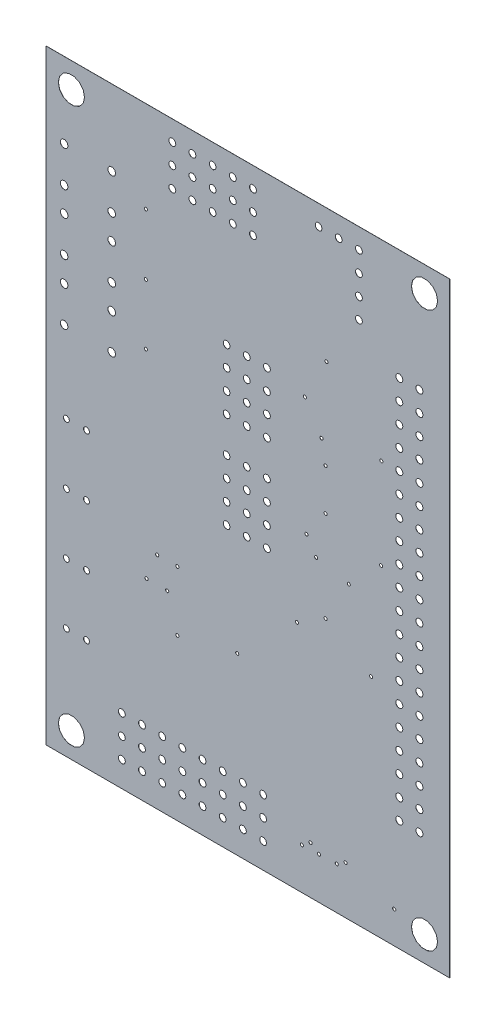
# Autodesk Inventor part: quick-start-plus_Outline4
Saved by Autodesk Inventor 2013 (Build 170138000, 138)
## iProperties
Created: 2013-01-27
Part Number: quick-start-plus_Outline4
Material: Generic
Document SubType Name: Modeling
Designer: davidgitz
Density: 1 g/cm^3
Author: davidgitz
Autodesk Inventor part; units mm, degrees
ref_plane "YZ Plane" through (0, 0, 0) normal (1, 0, 0) x (0, 1, 0)
ref_plane "XZ Plane" through (0, 0, 0) normal (0, 1, 0) x (-1, 0, 0)
ref_plane "XY Plane" through (0, 0, 0) normal (0, 0, 1) x (1, 0, 0)
sketch "Sketch1" plane through (0, 0, 0) normal (0, 0, 1) x (1, 0, 0)
  line L0 (203.2, 203.2) -> (254, 203.2)
  line L1 (254, 203.2) -> (254, 279.4)
  line L2 (254, 279.4) -> (203.2, 279.4)
  line L3 (203.2, 279.4) -> (203.2, 203.2)
  circle A0 centre (236.474, 209.1944) radius 0.2032
  circle A1 centre (227.2538, 225.2218) radius 0.2032
  circle A2 centre (219.71, 223.393) radius 0.2032
  circle A3 centre (237.1852, 240.6396) radius 0.2032
  circle A4 centre (238.379, 251.2314) radius 0.2032
  circle A5 centre (238.4806, 262.636) radius 0.2032
  circle A6 centre (237.871, 253.9746) radius 0.2032
  circle A7 centre (245.3894, 255.27) radius 0.2032
  circle A8 centre (245.364, 243.84) radius 0.2032
  circle A9 centre (235.966, 242.57) radius 0.2032
  circle A10 centre (234.7722, 232.3592) radius 0.2032
  circle A11 centre (244.094, 231.1146) radius 0.2032
  circle A12 centre (217.17, 230.9114) radius 0.2032
  circle A13 centre (219.71, 230.9114) radius 0.2032
  circle A14 centre (247.015, 207.2132) radius 0.2032
  circle A15 centre (215.7476, 267.8938) radius 0.2032
  circle A16 centre (215.7476, 260.223) radius 0.2032
  circle A17 centre (215.7476, 252.6284) radius 0.2032
  circle A18 centre (241.3, 239.776) radius 0.2032
  circle A19 centre (238.379, 234.569) radius 0.2032
  circle A20 centre (238.379, 246.0244) radius 0.2032
  circle A21 centre (235.7628, 257.429) radius 0.2032
  circle A22 centre (215.8238, 227.6602) radius 0.2032
  circle A23 centre (218.44, 227.6348) radius 0.2032
  circle A24 centre (240.8936, 209.2198) radius 0.2032
  circle A25 centre (239.776, 208.534) radius 0.2032
  circle A26 centre (237.5408, 208.4578) radius 0.2032
  circle A27 centre (235.3818, 208.407) radius 0.2032
  circle A28 centre (212.725, 211.455) radius 0.4445
  circle A29 centre (212.725, 208.915) radius 0.4445
  circle A30 centre (212.725, 206.375) radius 0.4445
  circle A31 centre (215.265, 211.455) radius 0.4445
  circle A32 centre (215.265, 208.915) radius 0.4445
  circle A33 centre (215.265, 206.375) radius 0.4445
  circle A34 centre (217.805, 211.455) radius 0.4445
  circle A35 centre (217.805, 208.915) radius 0.4445
  circle A36 centre (217.805, 206.375) radius 0.4445
  circle A37 centre (220.345, 211.455) radius 0.4445
  circle A38 centre (220.345, 208.915) radius 0.4445
  circle A39 centre (220.345, 206.375) radius 0.4445
  circle A40 centre (222.885, 211.455) radius 0.4445
  circle A41 centre (222.885, 208.915) radius 0.4445
  circle A42 centre (222.885, 206.375) radius 0.4445
  circle A43 centre (225.425, 211.455) radius 0.4445
  circle A44 centre (225.425, 208.915) radius 0.4445
  circle A45 centre (225.425, 206.375) radius 0.4445
  circle A46 centre (227.965, 211.455) radius 0.4445
  circle A47 centre (227.965, 208.915) radius 0.4445
  circle A48 centre (227.965, 206.375) radius 0.4445
  circle A49 centre (230.505, 211.455) radius 0.4445
  circle A50 centre (230.505, 208.915) radius 0.4445
  circle A51 centre (230.505, 206.375) radius 0.4445
  circle A52 centre (237.49, 276.86) radius 0.4445
  circle A53 centre (240.03, 276.86) radius 0.4445
  circle A54 centre (247.65, 265.43) radius 0.4572
  circle A55 centre (247.65, 262.89) radius 0.4572
  circle A56 centre (247.65, 260.35) radius 0.4572
  circle A57 centre (247.65, 257.81) radius 0.4572
  circle A58 centre (247.65, 255.27) radius 0.4572
  circle A59 centre (247.65, 252.73) radius 0.4572
  circle A60 centre (247.65, 250.19) radius 0.4572
  circle A61 centre (247.65, 247.65) radius 0.4572
  circle A62 centre (247.65, 245.11) radius 0.4572
  circle A63 centre (247.65, 242.57) radius 0.4572
  circle A64 centre (247.65, 240.03) radius 0.4572
  circle A65 centre (247.65, 237.49) radius 0.4572
  circle A66 centre (247.65, 234.95) radius 0.4572
  circle A67 centre (247.65, 232.41) radius 0.4572
  circle A68 centre (247.65, 229.87) radius 0.4572
  circle A69 centre (247.65, 227.33) radius 0.4572
  circle A70 centre (247.65, 224.79) radius 0.4572
  circle A71 centre (247.65, 222.25) radius 0.4572
  circle A72 centre (247.65, 219.71) radius 0.4572
  circle A73 centre (247.65, 217.17) radius 0.4572
  circle A74 centre (250.19, 217.17) radius 0.4572
  circle A75 centre (250.19, 219.71) radius 0.4572
  circle A76 centre (250.19, 222.25) radius 0.4572
  circle A77 centre (250.19, 224.79) radius 0.4572
  circle A78 centre (250.19, 227.33) radius 0.4572
  circle A79 centre (250.19, 229.87) radius 0.4572
  circle A80 centre (250.19, 232.41) radius 0.4572
  circle A81 centre (250.19, 234.95) radius 0.4572
  circle A82 centre (250.19, 237.49) radius 0.4572
  circle A83 centre (250.19, 240.03) radius 0.4572
  circle A84 centre (250.19, 242.57) radius 0.4572
  circle A85 centre (250.19, 245.11) radius 0.4572
  circle A86 centre (250.19, 247.65) radius 0.4572
  circle A87 centre (250.19, 250.19) radius 0.4572
  circle A88 centre (250.19, 252.73) radius 0.4572
  circle A89 centre (250.19, 255.27) radius 0.4572
  circle A90 centre (250.19, 257.81) radius 0.4572
  circle A91 centre (250.19, 260.35) radius 0.4572
  circle A92 centre (250.19, 262.89) radius 0.4572
  circle A93 centre (250.19, 265.43) radius 0.4572
  circle A94 centre (230.9876, 238.5314) radius 0.4445
  circle A95 centre (228.4476, 238.5314) radius 0.4445
  circle A96 centre (225.9076, 238.5314) radius 0.4445
  circle A97 centre (230.9876, 241.0714) radius 0.4445
  circle A98 centre (228.4476, 241.0714) radius 0.4445
  circle A99 centre (225.9076, 241.0714) radius 0.4445
  circle A100 centre (230.9876, 243.6114) radius 0.4445
  circle A101 centre (228.4476, 243.6114) radius 0.4445
  circle A102 centre (225.9076, 243.6114) radius 0.4445
  circle A103 centre (230.9876, 246.1514) radius 0.4445
  circle A104 centre (228.4476, 246.1514) radius 0.4445
  circle A105 centre (225.9076, 246.1514) radius 0.4445
  circle A106 centre (230.9876, 250.5964) radius 0.4445
  circle A107 centre (228.4476, 250.5964) radius 0.4445
  circle A108 centre (225.9076, 250.5964) radius 0.4445
  circle A109 centre (230.9876, 253.1364) radius 0.4445
  circle A110 centre (228.4476, 253.1364) radius 0.4445
  circle A111 centre (225.9076, 253.1364) radius 0.4445
  circle A112 centre (230.9876, 255.6764) radius 0.4445
  circle A113 centre (228.4476, 255.6764) radius 0.4445
  circle A114 centre (225.9076, 255.6764) radius 0.4445
  circle A115 centre (230.9876, 258.2164) radius 0.4445
  circle A116 centre (228.4476, 258.2164) radius 0.4445
  circle A117 centre (225.9076, 258.2164) radius 0.4445
  circle A118 centre (205.74, 217.17) radius 0.381
  circle A119 centre (208.28, 217.17) radius 0.381
  circle A120 centre (205.74, 224.79) radius 0.381
  circle A121 centre (208.28, 224.79) radius 0.381
  circle A122 centre (205.74, 232.41) radius 0.381
  circle A123 centre (208.28, 232.41) radius 0.381
  circle A124 centre (205.74, 240.03) radius 0.381
  circle A125 centre (208.28, 240.03) radius 0.381
  circle A126 centre (242.57, 269.24) radius 0.4445
  circle A127 centre (242.57, 271.78) radius 0.4445
  circle A128 centre (242.57, 274.32) radius 0.4445
  circle A129 centre (242.57, 276.86) radius 0.4445
  circle A130 centre (219.075, 271.78) radius 0.4445
  circle A131 centre (219.075, 274.32) radius 0.4445
  circle A132 centre (219.075, 276.86) radius 0.4445
  circle A133 centre (221.615, 271.78) radius 0.4445
  circle A134 centre (221.615, 274.32) radius 0.4445
  circle A135 centre (221.615, 276.86) radius 0.4445
  circle A136 centre (224.155, 271.78) radius 0.4445
  circle A137 centre (224.155, 274.32) radius 0.4445
  circle A138 centre (224.155, 276.86) radius 0.4445
  circle A139 centre (226.695, 271.78) radius 0.4445
  circle A140 centre (226.695, 274.32) radius 0.4445
  circle A141 centre (226.695, 276.86) radius 0.4445
  circle A142 centre (229.235, 271.78) radius 0.4445
  circle A143 centre (229.235, 274.32) radius 0.4445
  circle A144 centre (229.235, 276.86) radius 0.4445
  circle A145 centre (211.455, 262.255) radius 0.4953
  circle A146 centre (205.4606, 262.255) radius 0.4953
  circle A147 centre (205.4606, 257.7592) radius 0.4953
  circle A148 centre (211.455, 257.7592) radius 0.4953
  circle A149 centre (211.455, 269.875) radius 0.4953
  circle A150 centre (205.4606, 269.875) radius 0.4953
  circle A151 centre (205.4606, 265.3792) radius 0.4953
  circle A152 centre (211.455, 265.3792) radius 0.4953
  circle A153 centre (211.455, 254.635) radius 0.4953
  circle A154 centre (205.4606, 254.635) radius 0.4953
  circle A155 centre (205.4606, 250.1392) radius 0.4953
  circle A156 centre (211.455, 250.1392) radius 0.4953
  circle A157 centre (250.825, 206.375) radius 1.651
  circle A158 centre (250.825, 276.225) radius 1.651
  circle A159 centre (206.375, 276.225) radius 1.651
  circle A160 centre (206.375, 206.375) radius 1.651
  constraints: 161 centre point, 8 end point
extrude "quick-start-plus_Outline" add sketch "Sketch1" along normal blind 0.01
body "Solid1"
